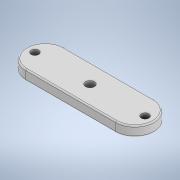
# Autodesk Inventor part: PropConnector
Saved by Autodesk Inventor 2022.1 (Build 261234020, 234B)
## iProperties
Created: 2022-10-16
Part Number: PropConnector
Material: Generic
Document SubType Name: Modeling
Designer: Alexander
Density: 1 g/cm^3
Appearance: Default
Author: Alexander
Autodesk Inventor part; units mm, degrees
ref_plane "YZ Plane" through (0, 0, 0) normal (1, 0, 0) x (0, 1, 0)
ref_plane "XZ Plane" through (0, 0, 0) normal (0, 1, 0) x (-1, 0, 0)
ref_plane "XY Plane" through (0, 0, 0) normal (0, 0, 1) x (1, 0, 0)
sketch "Sketch1" plane through (0, 0, 0) normal (0, 1, 0) x (-1, 0, 0)
  line L0 (25, -7.5) -> (-25, -7.5)
  line L1 (-25, -7.5) -> (-25, 7.5)
  line L2 (-25, 7.5) -> (25, 7.5)
  line L3 (25, 7.5) -> (25, -7.5)
  circle A0 centre (0, 0) radius 1.75
  circle A1 centre (-21.5, 0) radius 1.5
  line L4 (0, 11.4467) -> (0, -17.1004)
  circle A2 centre (21.5, 0) radius 1.5
  point P0 (0, -7.5)
  dimension "d0" = 15
  dimension "d1" = 50
  dimension "d2" = 25
  dimension "d3" = 3.5
  dimension "d4" = 7.5
  dimension "d7" = 3
  dimension "d9" = 7.5
  dimension "d10" = 2
  constraints: 10 end point, 3 centre point, 2 parallel, 1 coincident, 1 horizontal, 1 midpoint, 1 perpendicular, 1 symmetric about line, 1 vertical, 1 other
  measures "d0" distance of L0.end L1.end
  measures "d1" distance of L0.start L0.end
  measures "d2" distance from line of point (0, 0) L1
  measures "d3" diameter of A0
  measures "d4" distance of point (0, -7.5) point (0, 0)
  measures "d7" diameter of A1
  measures "d9" distance from line of L0 A1.centre
  measures "d10" distance edge to line of A1 L1
extrude "Extrusion2" add sketch "Sketch1" along normal blind 3.95 contours L0 L4 A0 L2 L3 | L0 L1 L2 L4 A0
fillet "Fillet1" radius 7.5 4 edges at (25, 1.975, 7.5) (25, 1.975, -7.5) (-25, 1.975, 7.5) (-25, 1.975, -7.5)
fillet "Fillet2" radius 0.5 8 edges at (22.8033, 3.95, 5.3033) (0, 3.95, -7.5) (-22.8033, 3.95, 5.3033) (0, 3.95, 7.5) (22.8033, 0, 5.3033) (0, 0, -7.5) (-22.8033, 0, 5.3033) (0, 0, 7.5)
body "Solid2"
